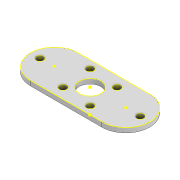
# Autodesk Inventor part: Motor_mount_plate
Saved by Autodesk Inventor 2022 (Build 260153000, 153)
## iProperties
Created: 2022-04-28
Part Number: Motor_mount_plate
Material: Generic
Document SubType Name: Modeling
Designer: dell
Density: 1 g/cm^3
Appearance: Default
Author: dell
Autodesk Inventor part; units mm, degrees
ref_plane "YZ Plane" through (0, 0, 0) normal (1, 0, 0) x (0, 1, 0)
ref_plane "XZ Plane" through (0, 0, 0) normal (0, 1, 0) x (-1, 0, 0)
ref_plane "XY Plane" through (0, 0, 0) normal (0, 0, 1) x (1, 0, 0)
sketch "Sketch2" plane through (0, 0, 0) normal (0, 1, 0) x (-1, 0, 0)
  line L0 (0, 0) -> (20, 0)
  line L1 (20, 0) -> (20, -20)
  line L2 (20, -20) -> (0, -20)
  line L3 (0, -20) -> (0, 0)
  line L4 (20, 0) -> (0, -20) construction
  line L5 (20, -20) -> (0, 0) construction
  circle A0 centre (15.6569, -4.3431) radius 1.5
  circle A1 centre (16.7175, -16.7175) radius 1.5
  circle A2 centre (3.2825, -3.2825) radius 1.5
  circle A3 centre (4.3431, -15.6569) radius 1.5
  circle A4 centre (10, -10) radius 4.5
  line L6 (20, -20) -> (25, -20)
  line L7 (25, -20) -> (25, 0)
  line L8 (25, 0) -> (20, 0)
  line L9 (20, 0) -> (20, -20)
  line L10 (0, -20) -> (-5, -20)
  line L11 (-5, -20) -> (-5, 0)
  line L12 (-5, 0) -> (0, 0)
  line L13 (0, 0) -> (0, -20)
  arc A5 (25, -20) -> (25, 0) centre (25, -10) ccw
  arc A6 (-5, 0) -> (-5, -20) centre (-5, -10) ccw
  circle A7 centre (31, -10) radius 1.5
  circle A8 centre (-11, -10) radius 1.5
  dimension "d37" = 3
  dimension "d38" = 3
  dimension "d39" = 3
  dimension "d40" = 3
  dimension "d41" = 9.5
  dimension "d42" = 9.5
  dimension "d43" = 8
  dimension "d44" = 8
  dimension "d60" = 20
  dimension "d61" = 9
  dimension "d66" = 5
  dimension "d67" = 5
  dimension "d68" = 3
  dimension "d69" = 3
  dimension "d70" = 6
  dimension "d71" = 6
  constraints: 28 end point, 9 centre point, 6 parallel, 4 perpendicular, 4 point on circle, 4 point on line, 4 tangent, 3 horizontal, 2 collinear, 1 coincident, 1 midpoint
  measures "d37" diameter of A0
  measures "d38" diameter of A1
  measures "d39" diameter of A2
  measures "d40" diameter of A3
  measures "d41" distance of point (10, -10) A2.centre
  measures "d42" distance of A1.centre point (10, -10)
  measures "d43" distance of A0.centre point (10, -10)
  measures "d44" distance of A3.centre point (10, -10)
  measures "d60" distance of L2.end L0.start
  measures "d61" diameter of A4
  measures "d66" distance of L7.end L8.end
  measures "d67" distance of L11.end L12.end
  measures "d68" diameter of A7
  measures "d69" diameter of A8
  measures "d70" distance of A5.centre A7.centre
  measures "d71" distance of A6.centre A8.centre
extrude "Extrusion2" add sketch "Sketch2" along normal blind 2
sketch "Sketch3" plane through (0, 2, 0) normal (0, 1, 0) x (1, 0, 0)
  line L0 (5, 20) -> (-25, 20) projected
  arc A0 (-25, 20) -> (-25, 0) centre (-25, 10) ccw projected
  line L1 (-25, 0) -> (5, 0) projected
  arc A1 (5, 0) -> (5, 20) centre (5, 10) ccw projected
  circle A2 centre (-16.7175, 16.7175) radius 1.5 projected
  circle A3 centre (-3.2825, 3.2825) radius 1.5 projected
  circle A4 centre (-10, 10) radius 4.5 projected
  circle A5 centre (-4.3431, 15.6569) radius 1.5 projected
  circle A6 centre (-15.6569, 4.3431) radius 1.5 projected
  circle A7 centre (-31, 10) radius 1.5 projected
  circle A8 centre (11, 10) radius 1.5 projected
  point P0 (0, 0)
body "Solid2"
